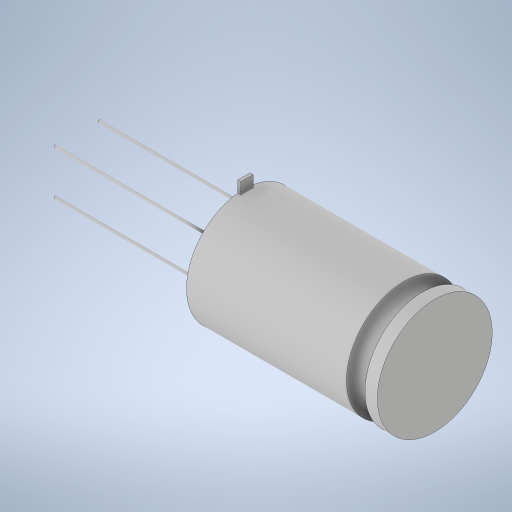
# Autodesk Inventor part: IR Sensor
Saved by Autodesk Inventor 2024 (Build 280153000, 153)
## iProperties
Created: 2024-01-19
Part Number: IR Sensor
Material: Generic
Document SubType Name: Modeling
Designer: student
Density: 1 g/cm^3
Appearance: Default
Author: student
Autodesk Inventor part; units mm, degrees
ref_plane "YZ Plane" through (0, 0, 0) normal (1, 0, 0) x (0, 1, 0)
ref_plane "XZ Plane" through (0, 0, 0) normal (0, 1, 0) x (-1, 0, 0)
ref_plane "XY Plane" through (0, 0, 0) normal (0, 0, 1) x (1, 0, 0)
sketch "Sketch1" plane through (0, 0, 0) normal (0, 1, 0) x (-1, 0, 0)
  circle A0 centre (0, 0) radius 4.65
  dimension "d0" = 9.3
  constraints: 1 centre point, 1 coincident
  measures "d0" diameter of A0
extrude "Extrusion1" add sketch "Sketch1" along normal blind 15.45
sketch "Sketch2" plane through (0, 0, 0) normal (1, 0, 0) x (0, 1, 0)
  line L0 (15.45, -4.65) -> (15.45, 4.65) projected
  line L1 (0, -4.65) -> (0, 4.65) projected
  line L2 (0, -4.65) -> (15.45, -4.65) projected
  line L3 (0, 4.65) -> (15.45, 4.65) projected
  line L4 (0, -4.65) -> (1, -4.65)
  arc A0 (2.5, -4.65) -> (1, -4.65) centre (1.75, -4.65) ccw
  line L5 (2.5, -4.65) -> (1, -4.65)
  line L6 (-3.09, 0) -> (18.54, 0) projected
  point P0 (0, 0)
  dimension "d3" = 1
  dimension "d4" = 1.5
  dimension "d5" = 0.75
  constraints: 4 end point, 2 point on circle, 2 point on line, 1 centre point, 1 collinear
  measures "d3" distance of L2.start L4.end
  measures "d4" distance of L4.end L5.start
  measures "d5" radius of A0
revolve "Revolution1" cut sketch "Sketch2" angle 360 about axis through (0, -10, 0) along (0, 1, 0) contours L2 A0
sketch "Sketch3" plane through (0, 15.45, 0) normal (0, 1, 0) x (1, 0, 0)
  circle A0 centre (0, 0) radius 4.65 projected
  line L0 (0, 0) -> (0, 4.65)
  line L1 (0, 5.55) -> (0.5, 5.55)
  line L2 (0, 5.55) -> (-0.5, 5.55)
  line L3 (-0.5, 5.55) -> (-0.5, 4.623)
  line L4 (0.5, 5.55) -> (0.5, 4.623)
  circle A1 centre (0, 0) radius 4.65 projected
  dimension "d7" = 0.9
  dimension "d8" = 0.5
  dimension "d9" = 0.5
  constraints: 10 end point, 3 point on circle, 2 horizontal, 1 parallel, 1 perpendicular, 1 point on line, 1 vertical
  measures "d7" distance of L0.end L1.start
  measures "d8" distance of L1.start L1.end
  measures "d9" distance of L1.start L2.end
extrude "Extrusion2" add sketch "Sketch3" against normal blind 0.25 contours A0 L3 L2 L1 L4
sketch "Sketch5" plane through (0, 15.45, 0) normal (0, 1, 0) x (1, 0, 0)
  arc A0 (-0.5, 4.623) -> (0.5, 4.623) centre (0, 0) ccw projected
  line L0 (0.5, 4.623) -> (0.5, 5.55) projected
  line L1 (0.5, 5.55) -> (-0.5, 5.55) projected
  line L2 (-0.5, 5.55) -> (-0.5, 4.623) projected
  line L3 (0, 0) -> (4.65, 0) construction
  line L4 (0, 0) -> (1.7961, 1.7961) construction
  circle A1 centre (1.781, 1.781) radius 0.1
  line L5 (1.781, 1.781) -> (1.781, 0) construction
  circle A2 centre (1.781, -1.781) radius 0.1
  line L6 (0, 0) -> (0, 5.55) construction
  circle A3 centre (-1.781, 1.781) radius 0.1
  circle A4 centre (-1.781, -1.781) radius 0.1
  circle A5 centre (-1.781, 1.781) radius 0.15
  dimension "d14" = 2.54
  dimension "d15" = 45
  dimension "d16" = 0.2
  dimension "d17" = 1.781
  dimension "d20" = 3.562
  dimension "d27" = 0.05
  constraints: 8 end point, 5 centre point, 2 point on line, 2 symmetric about line, 1 horizontal, 1 midpoint, 1 perpendicular, 1 point on circle, 1 vertical, 4 other
  measures "d14" distance of L3.start L4.end
  measures "d15" angle of L3 L4
  measures "d16" diameter of A1
  measures "d17" distance of L5.start L5.end
  measures "d20" distance of L5.start A2.centre
  measures "d27" radial gap between concentric circles of A3 A5
extrude "Extrusion3" add sketch "Sketch5" along normal blind 13.5 contours A1 | A2 | A3 | A4
extrude "Extrusion4" add sketch "Sketch5" along normal blind 0.25 contours A5
chamfer "Chamfer1" distance 0.05 angle 45 1 edges at (-1.931, 15.7, -1.781)
body "Solid1"
